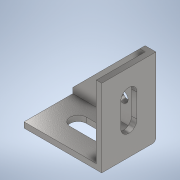
# Autodesk Inventor part: Sujetador2
Saved by Autodesk Inventor 2021 (Build 250183000, 183)
## iProperties
Created: 2020-11-09
Part Number: Sujetador2
Material: Acero, galvanizado
Document SubType Name: Modeling
Designer: juanm
Density: 7.85 g/cm^3
Appearance: Galvanizado
Author: juanm
Autodesk Inventor part; units mm, degrees
ref_plane "YZ Plane" through (0, 0, 0) normal (1, 0, 0) x (0, 1, 0)
ref_plane "XZ Plane" through (0, 0, 0) normal (0, 1, 0) x (-1, 0, 0)
ref_plane "XY Plane" through (0, 0, 0) normal (0, 0, 1) x (1, 0, 0)
sketch "Boceto1" plane through (0, 0, 0) normal (0, 0, 1) x (1, 0, 0)
  line L0 (49.5506, 21.8243) -> (55.5506, 21.8243)
  line L1 (55.5506, 21.8243) -> (55.5506, -21.1757)
  line L2 (55.5506, -21.1757) -> (12.5506, -21.1757)
  line L3 (12.5506, -21.1757) -> (12.5506, -15.1757)
  line L4 (55.5506, 21.8243) -> (49.5506, 21.8243)
  line L5 (12.5506, -21.1757) -> (12.5506, -15.1757)
  line L6 (12.5506, -15.1757) -> (49.5506, 21.8243)
  circle A0 centre (40.1551, -5.7801) radius 3
  point P0 (0, 0)
  dimension "d0" = 43
  dimension "d1" = 43
  dimension "d2" = 6
  dimension "d3" = 6
  dimension "d4" = 6
  constraints: 14 end point, 2 parallel, 1 centre point, 1 horizontal, 1 perpendicular
  measures "d0" distance of L1.end L2.end
  measures "d1" distance of L0.end L1.end
  measures "d2" distance of L0.start L0.end
  measures "d3" distance of L3.end L2.end
  measures "d4" diameter of A0
extrude "Extrusión1" add sketch "Boceto1" along normal blind 3
sketch "Boceto2" plane through (0, 0, 3) normal (0, 0, 1) x (1, 0, 0)
  line L0 (12.5506, -15.1757) -> (12.5506, -21.1757) projected
  line L1 (55.5506, -21.1757) -> (55.5506, 21.8243) projected
  line L2 (12.5506, -21.1757) -> (55.5506, -21.1757)
  line L3 (55.5506, -21.1757) -> (55.5506, -18.1757)
  line L4 (55.5506, -18.1757) -> (12.5506, -18.1757)
  line L5 (12.5506, -18.1757) -> (12.5506, -21.1757)
  point P0 (0, 0)
  dimension "d7" = 3
  constraints: 8 end point, 2 parallel, 1 horizontal, 1 perpendicular, 1 point on line
  measures "d7" distance of L3.end L2.end
extrude "Extrusión2" add sketch "Boceto2" along normal blind 27
sketch "Boceto3" plane through (0, 0, 3) normal (0, 0, 1) x (1, 0, 0)
  line L0 (12.5506, -18.1757) -> (55.5506, -18.1757) projected
  line L1 (55.5506, 21.8243) -> (49.5506, 21.8243) projected
  line L2 (55.5506, -18.1757) -> (52.5506, -18.1757)
  line L3 (52.5506, -18.1757) -> (52.5506, 21.8243)
  line L4 (52.5506, 21.8243) -> (55.5506, 21.8243)
  line L5 (55.5506, 21.8243) -> (55.5506, -18.1757)
  point P0 (0, 0)
  constraints: 8 end point, 2 parallel, 1 horizontal, 1 midpoint, 1 perpendicular
extrude "Extrusión3" add sketch "Boceto3" along normal blind 27
fillet "Empalme1" radius 2 1 edges at (34.0506, -21.1757, 0)
sketch "Boceto4" plane through (52.5506, -18.1757, 3) normal (-1, 0, 0) x (0, 0, 1)
  line L0 (-3, 40) -> (27, 40) projected
  line L1 (27, 40) -> (12, 40)
  line L2 (-1, -3) -> (27, -3) projected
  line L3 (16.5, 26) -> (16.5, 13)
  line L4 (7.5, 13) -> (7.5, 26)
  line L5 (27, 40) -> (27, 0) projected
  arc A0 (16.5, 26) -> (7.5, 26) centre (12, 26) ccw
  arc A1 (7.5, 13) -> (16.5, 13) centre (12, 13) ccw
  point P0 (-3, 18.1757)
  dimension "d13" = 15
  dimension "d15" = 9
  dimension "d16" = 13
  dimension "d19" = 9
  dimension "d20" = 9
  constraints: 6 end point, 4 point on circle, 2 centre point, 1 midpoint, 1 parallel
  measures "d13" distance of L0.end L1.end
  measures "d15" distance of L3.end L4.start
  measures "d16" distance of L3.start L3.end
  measures "d19" diameter of A0
  measures "d20" diameter of A1
extrude "Extrusión4" cut sketch "Boceto4" against normal blind 3
sketch "Boceto5" plane through (12.5506, -18.1757, 30) normal (0, 1, 0) x (1, 0, 0)
  line L0 (0, 30) -> (0, 15)
  line L1 (0, 28) -> (0, 0) projected
  line L2 (43, 19.5) -> (43, 10.5) projected
  line L3 (15, 10.5) -> (28, 10.5)
  line L4 (28, 19.5) -> (15, 19.5)
  line L5 (37, 30) -> (0, 30) projected
  arc A0 (15, 19.5) -> (15, 10.5) centre (15, 15) ccw
  arc A1 (28, 10.5) -> (28, 19.5) centre (28, 15) ccw
  point P0 (-12.5506, 30)
  dimension "d23" = 15
  dimension "d28" = 19.5
  constraints: 6 end point, 4 point on circle, 2 centre point, 1 horizontal, 1 parallel, 1 point on line
  measures "d23" distance of L0.start L0.end
  measures "d28" distance between parallel lines of L5 L3
extrude "Extrusión5" cut sketch "Boceto5" against normal blind 3
sketch "Boceto6" plane through (52.5506, -18.1757, 3) normal (-1, 0, 0) x (0, 0, 1)
  point P0 (-3, 18.1757)
